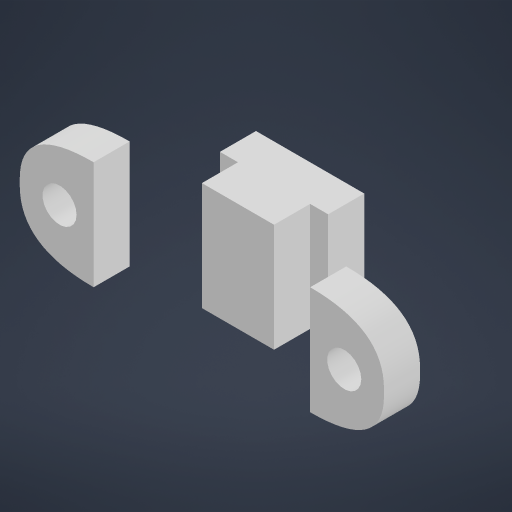
# Autodesk Inventor part: Connector_B
Saved by Autodesk Inventor 2024.1 (Build 281209000, 209)
## iProperties
Created: 2023-08-17
Part Number: Connector_B
Material: Generic
Document SubType Name: Modeling
Designer: Eleanor
Density: 1 g/cm^3
Appearance: Default
Author: Eleanor
Autodesk Inventor part; units mm, degrees
ref_plane "Work Plane7" through (0, 3.175, 0) normal (0, 1, 0) x (1, 0, 0)
ref_plane "Work Plane8" through (9.525, 0, -19.05) normal (0, 0, -1) x (-1, 0, 0)
sketch "Sketch4" plane through (9.525, 0, -19.05) normal (0, 0, -1) x (-1, 0, 0)
  line L0 (12.7, 0) -> (6.35, 0)
  line L1 (6.35, 0) -> (6.35, 9.525)
  line L2 (6.35, 9.525) -> (12.7, 9.525)
  line L3 (12.7, 9.525) -> (12.7, 0)
  line L4 (12.7, 0) -> (6.35, 9.525) construction
  line L5 (6.35, 0) -> (12.7, 9.525) construction
  point P0 (9.525, 0)
  point P1 (9.525, 4.7625)
  constraints: 12 end point, 2 midpoint, 2 parallel, 1 horizontal, 1 perpendicular
extrude "Extrusion4" add sketch "Sketch4" along normal blind 3.175
sketch "Sketch5" plane through (9.525, 0, -22.225) normal (0, 0, -1) x (-1, 0, 0)
  line L0 (4.7625, 0) -> (14.2875, 0)
  line L1 (14.2875, 0) -> (14.2875, 9.525)
  line L2 (14.2875, 9.525) -> (4.7625, 9.525)
  line L3 (4.7625, 9.525) -> (4.7625, 0)
  line L4 (4.7625, 0) -> (14.2875, 9.525) construction
  line L5 (14.2875, 0) -> (4.7625, 9.525) construction
  point P0 (9.525, 0)
  point P1 (9.525, 4.7625)
  constraints: 12 end point, 2 midpoint, 2 parallel, 1 horizontal, 1 perpendicular
extrude "Extrusion5" add sketch "Sketch5" along normal blind 3.175
ref_plane "Work Plane6" through (3.175, 9.525, 25.4) normal (0, 0, 1) x (1, 0, 0)
ref_plane "Work Plane5" through (-4.7625, 0, 3.175) normal (0, 0, 1) x (1, 0, 0)
sketch "Sketch8" plane through (9.525, 0, -19.05) normal (0, 0, 1) x (1, 0, 0)
  circle A0 centre (3, 4.7625) radius 1.5
  line L0 (6.5, 4.5085) -> (6.5, 5.0165)
  line L1 (6.5, 5.0165) -> (6.5, 9.525) construction
  line L2 (6.5, 9.525) -> (0, 9.525) construction
  spline S0 degree 2 poles (6.5, 5.0165) (6.5, 9.525) (0, 9.525) knots 1 1 1 2 2 2
  line L3 (6.5, 4.5085) -> (6.5, 0) construction
  line L4 (6.5, 0) -> (0, 0) construction
  spline S1 degree 2 poles (6.5, 4.5085) (6.5, 0) (0, 0) knots 1 1 1 2 2 2
  line L5 (-9.525, 0) -> (-9.525, 9.525)
  line L6 (-14.2875, 9.525) -> (-4.7625, 9.525)
  line L7 (0, 9.525) -> (0, 0)
  line L8 (0, 0) -> (0, 9.525)
  circle A1 centre (-22.05, 4.7625) radius 1.5
  line L9 (-25.55, 4.5085) -> (-25.55, 5.0165)
  line L10 (-25.55, 5.0165) -> (-25.55, 9.525) construction
  spline S2 degree 2 poles (-25.55, 5.0165) (-25.55, 9.525) (-19.05, 9.525) knots 1 1 1 2 2 2
  line L11 (-25.55, 9.525) -> (-19.05, 9.525) construction
  line L12 (-25.55, 4.5085) -> (-25.55, 0) construction
  spline S3 degree 2 poles (-25.55, 4.5085) (-25.55, 0) (-19.05, 0) knots 1 1 1 2 2 2
  line L13 (-25.55, 0) -> (-19.05, 0) construction
  line L14 (-19.05, 9.525) -> (-19.05, 0)
  line L15 (-19.05, 0) -> (-19.05, 9.525)
  point P0 (-9.525, 0)
  point P1 (4.5, 4.7625)
  point P2 (-23.55, 4.7625)
  dimension "d30" = 3
  constraints: 16 end point, 8 symmetric about line, 3 vertical, 2 horizontal alignment, 2 point on line, 1 horizontal, 1 midpoint, 16 other
extrude "Extrusion8" add sketch "Sketch8" along normal blind 3.175
body "Solid1"
